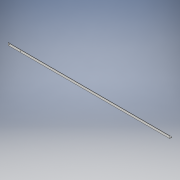
# Autodesk Inventor part: Upper Long L
Saved by Autodesk Inventor 2017 (Build 210142000, 142)
## iProperties
Created: 2018-08-22
Part Number: Upper Long L
Material: Generic
Document SubType Name: Modeling
Designer: sinner
Density: 1 g/cm^3
Appearance: Default
Author: sinner
Autodesk Inventor part; units mm, degrees
ref_plane "YZ Plane" through (0, 0, 0) normal (1, 0, 0) x (0, 1, 0)
ref_plane "XZ Plane" through (0, 0, 0) normal (0, 1, 0) x (-1, 0, 0)
ref_plane "XY Plane" through (0, 0, 0) normal (0, 0, 1) x (1, 0, 0)
sketch "Sketch1" plane through (0, 0, 0) normal (1, 0, 0) x (0, 1, 0)
  line L0 (0, 0) -> (25.4, 0)
  line L1 (3.2512, -25.4) -> (0, -25.4)
  line L2 (0, -25.4) -> (0, 0)
  line L3 (3.2512, -3.2512) -> (25.4, -3.2512)
  line L4 (3.2512, -25.4) -> (3.2512, -3.2512)
  line L5 (25.4, 0) -> (25.4, -3.2512)
  dimension "d0" = 25.4
  dimension "d1" = 3.2512
  constraints: 14 end point, 3 perpendicular, 2 horizontal, 2 parallel
  measures "d0" distance of L1.end L0.start
  measures "d1" distance of L1.start L1.end
extrude "Extrusion1" add sketch "Sketch1" along normal blind 1828.8
sketch "Sketch2" plane through (0, 0, 0) normal (0, 0, 1) x (1, 0, 0)
  line L0 (0, 0) -> (0, 25.4) projected
  line L1 (0, 12.7) -> (44.4361, 12.7) construction
  circle A0 centre (12.7, 12.7) radius 3.175
  circle A1 centre (139.7, 12.7) radius 3.175
  dimension "d4" = 6.35
  dimension "d5" = 12.7
  dimension "d6" = 139.7
  constraints: 2 centre point, 2 end point, 2 point on line, 1 equal radius, 1 horizontal, 1 midpoint
  measures "d4" diameter of A1
  measures "d5" distance from line of L0 A0.centre
  measures "d6" distance from line of L0 A1.centre
extrude "Extrusion2" cut sketch "Sketch2" against normal blind 1828.8
sketch "Sketch3" plane through (0, 0, -25.4) normal (0, -1, 0) x (1, 0, 0)
  line L0 (0, 0) -> (0, 25.4) projected
  line L1 (0, 12.7) -> (119.8367, 12.7) construction
  circle A0 centre (12.7, 12.7) radius 3.175
  circle A1 centre (139.7, 12.7) radius 3.175
  dimension "d9" = 6.35
  dimension "d10" = 12.7
  dimension "d11" = 139.7
  constraints: 2 centre point, 2 end point, 2 point on line, 1 equal radius, 1 horizontal, 1 midpoint
  measures "d9" diameter of A1
  measures "d10" distance from line of L0 A0.centre
  measures "d11" distance from line of L0 A1.centre
extrude "Extrusion3" cut sketch "Sketch3" against normal blind 1828.8
body "Solid1"
